Autodesk Fusion 360 part; units mm, degrees
note: some values were not read from the file. Set by a fixed rule: which sketch regions a step uses.
(part 2 of 2)
sketch "Sketch5" plane through (0, 0, 0) normal (0, -1, 0) x (1, 0, 0)
  line L0 (-69, 61.2598) -> (-1, 61.2598)
  line L1 (-1, 61.2598) -> (-1, 1.2598)
  line L2 (-1, 1.2598) -> (-69, 1.2598)
  line L3 (-69, 1.2598) -> (-69, 61.2598)
  line L4 (-1, 61.2598) -> (-69, 61.2598)
  spline S0 degree 2 poles (-53.1537, 11.7525) (-53.6706, 11.7525) (-54.074, 11.8908) knots 0 0 0 1 1 1
  spline S1 degree 2 poles (-54.074, 11.8908) (-54.4774, 12.029) (-54.7587, 12.3334) knots 0 0 0 1 1 1
  spline S2 degree 2 poles (-54.7587, 12.3334) (-55.0401, 12.6377) (-55.1595, 13.1862) knots 0 0 0 1 1 1
  line L5 (-55.1595, 13.1862) -> (-54.4168, 13.4427)
  spline S3 degree 2 poles (-54.4168, 13.4427) (-54.2643, 12.9203) (-53.9481, 12.7142) knots 0 0 0 1 1 1
  spline S4 degree 2 poles (-53.9481, 12.7142) (-53.632, 12.5081) (-53.1537, 12.5081) knots 0 0 0 1 1 1
  spline S5 degree 2 poles (-53.1537, 12.5081) (-52.5548, 12.5081) (-52.2487, 12.7585) knots 0 0 0 1 1 1
  spline S6 degree 2 poles (-52.2487, 12.7585) (-51.9425, 13.009) (-51.9425, 13.4888) knots 0 0 0 1 1 1
  line L6 (-51.9425, 13.4888) -> (-51.9425, 13.6757)
  spline S7 degree 2 poles (-51.9425, 13.6757) (-51.9425, 13.9799) (-52.0917, 14.1742) knots 0 0 0 1 1 1
  spline S8 degree 2 poles (-52.0917, 14.1742) (-52.2408, 14.3684) (-52.4867, 14.4882) knots 0 0 0 1 1 1
  spline S9 degree 2 poles (-52.4867, 14.4882) (-52.7327, 14.6081) (-53.1343, 14.7388) knots 0 0 0 1 1 1
  spline S10 degree 2 poles (-53.1343, 14.7388) (-53.1481, 14.7432) (-53.1611, 14.7476) knots 0 0 0 1 1 1
  spline S11 degree 2 poles (-53.1611, 14.7476) (-53.1741, 14.7519) (-53.1871, 14.7562) knots 0 0 0 1 1 1
  line L7 (-53.1871, 14.7562) -> (-53.287, 14.7912)
  spline S12 degree 2 poles (-53.287, 14.7912) (-53.839, 14.96) (-54.1806, 15.124) knots 0 0 0 1 1 1
  spline S13 degree 2 poles (-54.1806, 15.124) (-54.5222, 15.288) (-54.7648, 15.6136) knots 0 0 0 1 1 1
  spline S14 degree 2 poles (-54.7648, 15.6136) (-55.0074, 15.9393) (-55.0074, 16.4797) knots 0 0 0 1 1 1
  line L8 (-55.0074, 16.4797) -> (-55.0074, 16.6362)
  spline S15 degree 2 poles (-55.0074, 16.6362) (-55.0074, 17.2009) (-54.7773, 17.5897) knots 0 0 0 1 1 1
  spline S16 degree 2 poles (-54.7773, 17.5897) (-54.5471, 17.9786) (-54.1035, 18.1799) knots 0 0 0 1 1 1
  spline S17 degree 2 poles (-54.1035, 18.1799) (-53.6598, 18.3812) (-53.032, 18.3812) knots 0 0 0 1 1 1
  spline S18 degree 2 poles (-53.032, 18.3812) (-52.5442, 18.3812) (-52.1831, 18.2423) knots 0 0 0 1 1 1
  spline S19 degree 2 poles (-52.1831, 18.2423) (-51.8221, 18.1034) (-51.5874, 17.8159) knots 0 0 0 1 1 1
  spline S20 degree 2 poles (-51.5874, 17.8159) (-51.3526, 17.5283) (-51.2261, 17.0037) knots 0 0 0 1 1 1
  line L9 (-51.2261, 17.0037) -> (-51.9597, 16.7518)
  spline S21 degree 2 poles (-51.9597, 16.7518) (-52.1233, 17.2447) (-52.3733, 17.4351) knots 0 0 0 1 1 1
  spline S22 degree 2 poles (-52.3733, 17.4351) (-52.6233, 17.6256) (-53.032, 17.6256) knots 0 0 0 1 1 1
  spline S23 degree 2 poles (-53.032, 17.6256) (-53.6144, 17.6256) (-53.9113, 17.3782) knots 0 0 0 1 1 1
  spline S24 degree 2 poles (-53.9113, 17.3782) (-54.2083, 17.1307) (-54.2083, 16.6623) knots 0 0 0 1 1 1
  line L10 (-54.2083, 16.6623) -> (-54.2083, 16.5058)
  spline S25 degree 2 poles (-54.2083, 16.5058) (-54.2083, 16.2013) (-54.0419, 16.0134) knots 0 0 0 1 1 1
  spline S26 degree 2 poles (-54.0419, 16.0134) (-53.8756, 15.8255) (-53.6159, 15.7142) knots 0 0 0 1 1 1
  spline S27 degree 2 poles (-53.6159, 15.7142) (-53.3562, 15.6029) (-52.8894, 15.459) knots 0 0 0 1 1 1
  spline S28 degree 2 poles (-52.8894, 15.459) (-52.8716, 15.4555) (-52.8485, 15.4488) knots 0 0 0 1 1 1
  spline S29 degree 2 poles (-52.8485, 15.4488) (-52.8254, 15.4422) (-52.8153, 15.4354) knots 0 0 0 1 1 1
  spline S30 degree 2 poles (-52.8153, 15.4354) (-52.8034, 15.4331) (-52.7835, 15.4251) knots 0 0 0 1 1 1
  spline S31 degree 2 poles (-52.7835, 15.4251) (-52.7635, 15.4171) (-52.7424, 15.4118) knots 0 0 0 1 1 1
  spline S32 degree 2 poles (-52.7424, 15.4118) (-52.262, 15.262) (-51.9272, 15.0798) knots 0 0 0 1 1 1
  spline S33 degree 2 poles (-51.9272, 15.0798) (-51.5925, 14.8976) (-51.368, 14.5597) knots 0 0 0 1 1 1
  spline S34 degree 2 poles (-51.368, 14.5597) (-51.1435, 14.2218) (-51.1435, 13.7018) knots 0 0 0 1 1 1
  line L11 (-51.1435, 13.7018) -> (-51.1435, 13.4975)
  spline S35 degree 2 poles (-51.1435, 13.4975) (-51.1435, 12.9348) (-51.3763, 12.5429) knots 0 0 0 1 1 1
  spline S36 degree 2 poles (-51.3763, 12.5429) (-51.6092, 12.1509) (-52.0603, 11.9517) knots 0 0 0 1 1 1
  spline S37 degree 2 poles (-52.0603, 11.9517) (-52.5113, 11.7525) (-53.1537, 11.7525) knots 0 0 0 1 1 1
  spline S38 degree 2 poles (-48.5484, 11.7525) (-49.0996, 11.7525) (-49.4991, 11.9706) knots 0 0 0 1 1 1
  spline S39 degree 2 poles (-49.4991, 11.9706) (-49.8986, 12.1887) (-50.1068, 12.6053) knots 0 0 0 1 1 1
  spline S40 degree 2 poles (-50.1068, 12.6053) (-50.3151, 13.0218) (-50.3151, 13.6018) knots 0 0 0 1 1 1
  line L12 (-50.3151, 13.6018) -> (-50.3151, 14.6365)
  spline S41 degree 2 poles (-50.3151, 14.6365) (-50.3151, 15.2443) (-50.1148, 15.6789) knots 0 0 0 1 1 1
  spline S42 degree 2 poles (-50.1148, 15.6789) (-49.9146, 16.1135) (-49.5275, 16.3453) knots 0 0 0 1 1 1
  spline S43 degree 2 poles (-49.5275, 16.3453) (-49.1404, 16.5771) (-48.6049, 16.5771) knots 0 0 0 1 1 1
  spline S44 degree 2 poles (-48.6049, 16.5771) (-48.0838, 16.5771) (-47.7085, 16.3547) knots 0 0 0 1 1 1
  spline S45 degree 2 poles (-47.7085, 16.3547) (-47.3333, 16.1323) (-47.1379, 15.7139) knots 0 0 0 1 1 1
  spline S46 degree 2 poles (-47.1379, 15.7139) (-46.9424, 15.2954) (-46.9424, 14.7147) knots 0 0 0 1 1 1
  line L13 (-46.9424, 14.7147) -> (-46.9424, 13.8088)
  line L14 (-46.9424, 13.8088) -> (-49.9108, 13.8088)
  line L15 (-49.9108, 13.8088) -> (-49.9108, 14.56)
  line L16 (-49.9108, 14.56) -> (-47.7285, 14.56)
  line L17 (-47.7285, 14.56) -> (-47.7285, 14.7538)
  spline S47 degree 2 poles (-47.7285, 14.7538) (-47.7285, 15.2667) (-47.9582, 15.5419) knots 0 0 0 1 1 1
  spline S48 degree 2 poles (-47.9582, 15.5419) (-48.1879, 15.8172) (-48.6049, 15.8172) knots 0 0 0 1 1 1
  spline S49 degree 2 poles (-48.6049, 15.8172) (-49.046, 15.8172) (-49.2875, 15.5281) knots 0 0 0 1 1 1
  spline S50 degree 2 poles (-49.2875, 15.5281) (-49.529, 15.2391) (-49.529, 14.6843) knots 0 0 0 1 1 1
  line L18 (-49.529, 14.6843) -> (-49.529, 13.5845)
  spline S51 degree 2 poles (-49.529, 13.5845) (-49.529, 13.0651) (-49.2744, 12.7887) knots 0 0 0 1 1 1
  spline S52 degree 2 poles (-49.2744, 12.7887) (-49.0197, 12.5124) (-48.5484, 12.5124) knots 0 0 0 1 1 1
  spline S53 degree 2 poles (-48.5484, 12.5124) (-48.2474, 12.5124) (-48.0407, 12.6606) knots 0 0 0 1 1 1
  spline S54 degree 2 poles (-48.0407, 12.6606) (-47.834, 12.8087) (-47.7307, 13.1427) knots 0 0 0 1 1 1
  line L19 (-47.7307, 13.1427) -> (-46.9946, 12.9239)
  spline S55 degree 2 poles (-46.9946, 12.9239) (-47.1266, 12.3237) (-47.5353, 12.0381) knots 0 0 0 1 1 1
  spline S56 degree 2 poles (-47.5353, 12.0381) (-47.944, 11.7525) (-48.5484, 11.7525) knots 0 0 0 1 1 1
  line L20 (-45.9898, 16.5075) -> (-45.1821, 16.5075)
  line L21 (-45.1821, 16.5075) -> (-45.1821, 11.8177)
  line L22 (-45.1821, 11.8177) -> (-45.9898, 11.8177)
  line L23 (-45.9898, 11.8177) -> (-45.9898, 16.5075)
  spline S57 degree 2 poles (-43.4249, 14.8669) (-43.4249, 15.3398) (-43.6502, 15.5807) knots 0 0 0 1 1 1
  spline S58 degree 2 poles (-43.6502, 15.5807) (-43.8754, 15.8215) (-44.3144, 15.8215) knots 0 0 0 1 1 1
  spline S59 degree 2 poles (-44.3144, 15.8215) (-44.7376, 15.8215) (-44.9598, 15.5877) knots 0 0 0 1 1 1
  spline S60 degree 2 poles (-44.9598, 15.5877) (-45.1821, 15.3538) (-45.1821, 14.8042) knots 0 0 0 1 1 1
  line L24 (-45.1821, 14.8042) -> (-45.4551, 15.6682)
  spline S61 degree 2 poles (-45.4551, 15.6682) (-45.2369, 16.1446) (-44.8814, 16.363) knots 0 0 0 1 1 1
  spline S62 degree 2 poles (-44.8814, 16.363) (-44.5259, 16.5814) (-44.0536, 16.5814) knots 0 0 0 1 1 1
  spline S63 degree 2 poles (-44.0536, 16.5814) (-43.3534, 16.5814) (-42.9853, 16.1364) knots 0 0 0 1 1 1
  spline S64 degree 2 poles (-42.9853, 16.1364) (-42.6172, 15.6914) (-42.6172, 14.8712) knots 0 0 0 1 1 1
  line L25 (-42.6172, 14.8712) -> (-42.6172, 11.8177)
  line L26 (-42.6172, 11.8177) -> (-43.4249, 11.8177)
  line L27 (-43.4249, 11.8177) -> (-43.4249, 14.8669)
  spline S65 degree 2 poles (-39.1259, 14.9886) (-39.1259, 15.4081) (-39.3483, 15.6344) knots 0 0 0 1 1 1
  spline S66 degree 2 poles (-39.3483, 15.6344) (-39.5707, 15.8607) (-39.9893, 15.8607) knots 0 0 0 1 1 1
  spline S67 degree 2 poles (-39.9893, 15.8607) (-40.2831, 15.8607) (-40.5059, 15.7226) knots 0 0 0 1 1 1
  spline S68 degree 2 poles (-40.5059, 15.7226) (-40.7287, 15.5846) (-40.8666, 15.2781) knots 0 0 0 1 1 1
  line L28 (-40.8666, 15.2781) -> (-41.5386, 15.4618)
  spline S69 degree 2 poles (-41.5386, 15.4618) (-41.4007, 16.0397) (-40.9932, 16.3105) knots 0 0 0 1 1 1
  spline S70 degree 2 poles (-40.9932, 16.3105) (-40.5858, 16.5814) (-39.9893, 16.5814) knots 0 0 0 1 1 1
  spline S71 degree 2 poles (-39.9893, 16.5814) (-39.4765, 16.5814) (-39.1031, 16.3935) knots 0 0 0 1 1 1
  spline S72 degree 2 poles (-39.1031, 16.3935) (-38.7296, 16.2056) (-38.5347, 15.853) knots 0 0 0 1 1 1
  spline S73 degree 2 poles (-38.5347, 15.853) (-38.3398, 15.5004) (-38.3398, 15.0104) knots 0 0 0 1 1 1
  line L29 (-38.3398, 15.0104) -> (-38.3398, 11.8177)
  line L30 (-38.3398, 11.8177) -> (-39.1259, 11.8177)
  line L31 (-39.1259, 11.8177) -> (-39.1259, 14.9886)
  spline S74 degree 2 poles (-40.1849, 11.7525) (-40.9119, 11.7525) (-41.3035, 12.1185) knots 0 0 0 1 1 1
  spline S75 degree 2 poles (-41.3035, 12.1185) (-41.6951, 12.4845) (-41.6951, 13.1714) knots 0 0 0 1 1 1
  spline S76 degree 2 poles (-41.6951, 13.1714) (-41.6951, 13.908) (-41.2968, 14.297) knots 0 0 0 1 1 1
  spline S77 degree 2 poles (-41.2968, 14.297) (-40.8984, 14.686) (-40.1501, 14.686) knots 0 0 0 1 1 1
  line L32 (-40.1501, 14.686) -> (-38.9157, 14.686)
  line L33 (-38.9157, 14.686) -> (-38.8441, 13.9913)
  line L34 (-38.8441, 13.9913) -> (-40.1458, 13.9913)
  spline S78 degree 2 poles (-40.1458, 13.9913) (-40.5299, 13.9913) (-40.7238, 13.7878) knots 0 0 0 1 1 1
  spline S79 degree 2 poles (-40.7238, 13.7878) (-40.9178, 13.5843) (-40.9178, 13.1714) knots 0 0 0 1 1 1
  spline S80 degree 2 poles (-40.9178, 13.1714) (-40.9178, 12.8181) (-40.7062, 12.637) knots 0 0 0 1 1 1
  spline S81 degree 2 poles (-40.7062, 12.637) (-40.4946, 12.4559) (-40.0675, 12.4559) knots 0 0 0 1 1 1
  spline S82 degree 2 poles (-40.0675, 12.4559) (-39.5922, 12.4559) (-39.3591, 12.605) knots 0 0 0 1 1 1
  spline S83 degree 2 poles (-39.3591, 12.605) (-39.1259, 12.754) (-39.1259, 13.121) knots 0 0 0 1 1 1
  line L35 (-39.1259, 13.121) -> (-38.8528, 12.5424)
  spline S84 degree 2 poles (-38.8528, 12.5424) (-38.9331, 12.2718) (-39.1147, 12.0975) knots 0 0 0 1 1 1
  spline S85 degree 2 poles (-39.1147, 12.0975) (-39.2963, 11.9231) (-39.566, 11.8378) knots 0 0 0 1 1 1
  spline S86 degree 2 poles (-39.566, 11.8378) (-39.8356, 11.7525) (-40.1849, 11.7525) knots 0 0 0 1 1 1
  line L36 (-40.4344, 17.5565) -> (-39.2062, 19.2071)
  line L37 (-39.2062, 19.2071) -> (-38.592, 18.7398)
  line L38 (-38.592, 18.7398) -> (-39.9084, 17.1779)
  line L39 (-39.9084, 17.1779) -> (-40.4344, 17.5565)
  line L40 (-37.2818, 16.5075) -> (-36.474, 16.5075)
  line L41 (-36.474, 16.5075) -> (-36.474, 11.8177)
  line L42 (-36.474, 11.8177) -> (-37.2818, 11.8177)
  line L43 (-37.2818, 11.8177) -> (-37.2818, 16.5075)
  spline S87 degree 2 poles (-34.7169, 14.8669) (-34.7169, 15.3398) (-34.9421, 15.5807) knots 0 0 0 1 1 1
  spline S88 degree 2 poles (-34.9421, 15.5807) (-35.1673, 15.8215) (-35.6064, 15.8215) knots 0 0 0 1 1 1
  spline S89 degree 2 poles (-35.6064, 15.8215) (-36.0296, 15.8215) (-36.2518, 15.5877) knots 0 0 0 1 1 1
  spline S90 degree 2 poles (-36.2518, 15.5877) (-36.474, 15.3538) (-36.474, 14.8042) knots 0 0 0 1 1 1
  line L44 (-36.474, 14.8042) -> (-36.747, 15.6682)
  spline S91 degree 2 poles (-36.747, 15.6682) (-36.5288, 16.1446) (-36.1733, 16.363) knots 0 0 0 1 1 1
  spline S92 degree 2 poles (-36.1733, 16.363) (-35.8179, 16.5814) (-35.3455, 16.5814) knots 0 0 0 1 1 1
  spline S93 degree 2 poles (-35.3455, 16.5814) (-34.6453, 16.5814) (-34.2772, 16.1364) knots 0 0 0 1 1 1
  spline S94 degree 2 poles (-34.2772, 16.1364) (-33.9091, 15.6914) (-33.9091, 14.8712) knots 0 0 0 1 1 1
  line L45 (-33.9091, 14.8712) -> (-33.9091, 11.8177)
  line L46 (-33.9091, 11.8177) -> (-34.7169, 11.8177)
  line L47 (-34.7169, 11.8177) -> (-34.7169, 14.8669)
  line L48 (-28.2981, 18.316) -> (-27.4903, 18.316)
  line L49 (-27.4903, 18.316) -> (-27.4903, 11.8177)
  line L50 (-27.4903, 11.8177) -> (-28.2981, 11.8177)
  line L51 (-28.2981, 11.8177) -> (-28.2981, 18.316)
  spline S95 degree 2 poles (-29.3876, 11.7482) (-29.8361, 11.7482) (-30.1604, 11.9488) knots 0 0 0 1 1 1
  spline S96 degree 2 poles (-30.1604, 11.9488) (-30.4846, 12.1494) (-30.652, 12.5256) knots 0 0 0 1 1 1
  spline S97 degree 2 poles (-30.652, 12.5256) (-30.8195, 12.9019) (-30.8195, 13.4236) knots 0 0 0 1 1 1
  line L52 (-30.8195, 13.4236) -> (-30.8195, 14.8712)
  spline S98 degree 2 poles (-30.8195, 14.8712) (-30.8195, 15.4027) (-30.6544, 15.7858) knots 0 0 0 1 1 1
  spline S99 degree 2 poles (-30.6544, 15.7858) (-30.4892, 16.1688) (-30.1704, 16.3751) knots 0 0 0 1 1 1
  spline S100 degree 2 poles (-30.1704, 16.3751) (-29.8515, 16.5814) (-29.4093, 16.5814) knots 0 0 0 1 1 1
  spline S101 degree 2 poles (-29.4093, 16.5814) (-28.958, 16.5814) (-28.6018, 16.3649) knots 0 0 0 1 1 1
  spline S102 degree 2 poles (-28.6018, 16.3649) (-28.2455, 16.1484) (-28.0251, 15.6943) knots 0 0 0 1 1 1
  line L53 (-28.0251, 15.6943) -> (-28.2981, 14.8478)
  spline S103 degree 2 poles (-28.2981, 14.8478) (-28.2981, 15.2016) (-28.3988, 15.4089) knots 0 0 0 1 1 1
  spline S104 degree 2 poles (-28.3988, 15.4089) (-28.4995, 15.6161) (-28.6927, 15.7384) knots 0 0 0 1 1 1
  spline S105 degree 2 poles (-28.6927, 15.7384) (-28.886, 15.8607) (-29.1484, 15.8607) knots 0 0 0 1 1 1
  spline S106 degree 2 poles (-29.1484, 15.8607) (-29.5606, 15.8607) (-29.7862, 15.6037) knots 0 0 0 1 1 1
  spline S107 degree 2 poles (-29.7862, 15.6037) (-30.0117, 15.3468) (-30.0117, 14.8625) knots 0 0 0 1 1 1
  line L54 (-30.0117, 14.8625) -> (-30.0117, 13.4236)
  spline S108 degree 2 poles (-30.0117, 13.4236) (-30.0117, 12.9605) (-29.7874, 12.7147) knots 0 0 0 1 1 1
  spline S109 degree 2 poles (-29.7874, 12.7147) (-29.563, 12.4689) (-29.1484, 12.4689) knots 0 0 0 1 1 1
  spline S110 degree 2 poles (-29.1484, 12.4689) (-28.8838, 12.4689) (-28.6917, 12.5904) knots 0 0 0 1 1 1
  spline S111 degree 2 poles (-28.6917, 12.5904) (-28.4996, 12.712) (-28.3989, 12.9214) knots 0 0 0 1 1 1
  spline S112 degree 2 poles (-28.3989, 12.9214) (-28.2981, 13.1308) (-28.2981, 13.4775) knots 0 0 0 1 1 1
  line L55 (-28.2981, 13.4775) -> (-28.0555, 12.6025)
  spline S113 degree 2 poles (-28.0555, 12.6025) (-28.2211, 12.1641) (-28.5645, 11.9561) knots 0 0 0 1 1 1
  spline S114 degree 2 poles (-28.5645, 11.9561) (-28.908, 11.7482) (-29.3876, 11.7482) knots 0 0 0 1 1 1
  line L56 (-26.6235, 18.316) -> (-25.8157, 18.316)
  line L57 (-25.8157, 18.316) -> (-25.8157, 15.9215)
  line L58 (-25.8157, 15.9215) -> (-26.6235, 15.9215)
  line L59 (-26.6235, 15.9215) -> (-26.6235, 18.316)
  line L60 (-23.5042, 18.316) -> (-22.6114, 18.316)
  line L61 (-22.6114, 18.316) -> (-20.6925, 11.8177)
  line L62 (-20.6925, 11.8177) -> (-21.5492, 11.8177)
  line L63 (-21.5492, 11.8177) -> (-23.0578, 17.4605)
  line L64 (-23.0578, 17.4605) -> (-24.5663, 11.8177)
  line L65 (-24.5663, 11.8177) -> (-25.4215, 11.8177)
  line L66 (-25.4215, 11.8177) -> (-23.5042, 18.316)
  line L67 (-24.2963, 13.9348) -> (-21.7393, 13.9348)
  line L68 (-21.7393, 13.9348) -> (-21.7393, 13.5297)
  line L69 (-21.7393, 13.5297) -> (-24.2963, 13.5297)
  line L70 (-24.2963, 13.5297) -> (-24.2963, 13.9348)
  line L71 (-20.0342, 16.5075) -> (-19.2264, 16.5075)
  line L72 (-19.2264, 16.5075) -> (-19.2264, 11.8177)
  line L73 (-19.2264, 11.8177) -> (-20.0342, 11.8177)
  line L74 (-20.0342, 11.8177) -> (-20.0342, 16.5075)
  spline S115 degree 2 poles (-17.547, 15.6737) (-17.7089, 15.7589) (-17.801, 15.7902) knots 0 0 0 1 1 1
  spline S116 degree 2 poles (-17.801, 15.7902) (-17.8931, 15.8215) (-18.0196, 15.8215) knots 0 0 0 1 1 1
  spline S117 degree 2 poles (-18.0196, 15.8215) (-18.5835, 15.8215) (-18.8976, 15.5435) knots 0 0 0 1 1 1
  spline S118 degree 2 poles (-18.8976, 15.5435) (-19.2116, 15.2654) (-19.2702, 14.6739) knots 0 0 0 1 1 1
  line L75 (-19.2702, 14.6739) -> (-19.4994, 15.6524)
  spline S119 degree 2 poles (-19.4994, 15.6524) (-19.2231, 16.1054) (-18.8021, 16.3434) knots 0 0 0 1 1 1
  spline S120 degree 2 poles (-18.8021, 16.3434) (-18.3811, 16.5814) (-17.8805, 16.5814) knots 0 0 0 1 1 1
  spline S121 degree 2 poles (-17.8805, 16.5814) (-17.7071, 16.5814) (-17.5667, 16.5297) knots 0 0 0 1 1 1
  spline S122 degree 2 poles (-17.5667, 16.5297) (-17.4263, 16.478) (-17.2875, 16.3384) knots 0 0 0 1 1 1
  line L76 (-17.2875, 16.3384) -> (-17.547, 15.6737)
  spline S123 degree 2 poles (-15.4109, 11.796) (-16.0009, 11.796) (-16.2784, 12.1257) knots 0 0 0 1 1 1
  spline S124 degree 2 poles (-16.2784, 12.1257) (-16.5559, 12.4554) (-16.5559, 13.0802) knots 0 0 0 1 1 1
  line L77 (-16.5559, 13.0802) -> (-16.5559, 17.8204)
  line L78 (-16.5559, 17.8204) -> (-15.7481, 17.8204)
  line L79 (-15.7481, 17.8204) -> (-15.7481, 13.0714)
  spline S125 degree 2 poles (-15.7481, 13.0714) (-15.7481, 12.8094) (-15.6425, 12.6827) knots 0 0 0 1 1 1
  spline S126 degree 2 poles (-15.6425, 12.6827) (-15.5368, 12.5559) (-15.3239, 12.5559) knots 0 0 0 1 1 1
  line L80 (-15.3239, 12.5559) -> (-14.8483, 12.5559)
  line L81 (-14.8483, 12.5559) -> (-14.8483, 11.796)
  line L82 (-14.8483, 11.796) -> (-15.4109, 11.796)
  line L83 (-17.0211, 16.5075) -> (-14.8483, 16.5075)
  line L84 (-14.8483, 16.5075) -> (-14.8483, 15.7694)
  line L85 (-14.8483, 15.7694) -> (-17.0211, 15.7694)
  line L86 (-17.0211, 15.7694) -> (-17.0211, 16.5075)
  point P0 (-69, 61.2598)
  point P1 (-1, 1.2598)
  constraint horizontal L0
  constraint vertical L1
  constraint horizontal L2
  constraint vertical L3
  constraint coincident P1 L1.end
  constraint coincident P0 L0.start
extrude "Extrude6" cut sketch "Sketch5" against normal up to surface (2 mm away) contours S0 S1 S2 L5 S3 S4 S5 S6 L6 S7 S8 S9 S10 S11 L7 S12 S13 S14 L8 S15 S16 S17 S18 S19 S20 L9 S21 S22 S23 S24 L10 S25 S26 S27 S28 S29 S30 S31 S32 S33 S34 L11 S35 S36 S37 | L14 L15 L16 L18 | S38 S39 S40 L12 S41 S42 S43 S44 S45 S46 L13 L14 L18 S51 S52 S53 S54 L19 S55 S56 | L20 L21 L22 L23 L24 S61 | L21 S57 S58 S59 S60 S61 S62 S63 S64 L25 L26 L27 | L21 L24 S61 | S65 S66 S67 S68 L28 S69 S70 S71 S72 S73 L29 L30 L31 L32 L33 L34 L35 S84 S85 | L31 L32 L33 L34 | L31 S74 S75 S76 S77 L32 L34 S78 S79 S80 S81 S82 S83 S85 S86 | L31 L35 S84 S85 | L36 L37 L38 L39 | L40 L41 L42 L43 L44 S91 | L41 S87 S88 S89 S90 S91 S92 S93 S94 L45 L46 L47 | L41 L44 S91 | L48 L49 L50 L51 S102 L53 L55 S113 | L51 S102 L53 | L51 S95 S96 S97 L52 S98 S99 S100 S101 S102 S103 S104 S105 S106 S107 L54 S108 S109 S110 S111 S112 S113 S114 | L51 L55 S113 | L56 L57 L58 L59 | L60 L61 L62 L63 L64 L65 L66 L67 L68 L69 L70 | L64 L67 L69 L70 | L63 L64 L67 L69 | L63 L67 L68 L69 | L71 L72 L73 L74 S118 L75 S119 | L72 S115 S116 S117 S118 S119 S120 S121 S122 L76 | L72 S118 L75 S119 | S123 S124 L77 L79 S125 S126 L80 L81 L82 L85 | L77 L83 L85 L86 | L77 L79 L83 L85 | L77 L78 L79 L83 | L79 L83 L84 L85
scale "Scale1" [suppressed]
equation "d25 = ( 13 / 2 ) * 1 mm"
equation "d26 = d24 / 2"
equation "d50 = ( ( 68 / 2 ) / 5 ) * 1 mm"
equation "d51 = d50"
equation "d52 = d50"
equation "d53 = d50"
